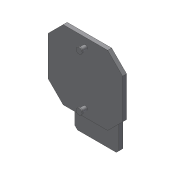
# Autodesk Inventor part: Maker-Bot-Raspberry-Pi-Holder
Saved by Autodesk Inventor 2015 (Build 190159000, 159)
## iProperties
Created: 2017-01-17
Part Number: Maker-Bot-Raspberry-Pi-Holder
Material: Generic
Document SubType Name: Modeling
Designer: Ghassan Yusuf
Density: 1 g/cm^3
Appearance: Default
Author: Ghassan Yusuf
Autodesk Inventor part; units mm, degrees
ref_plane "YZ Plane" through (0, 0, 0) normal (1, 0, 0) x (0, 1, 0)
ref_plane "XZ Plane" through (0, 0, 0) normal (0, 1, 0) x (-1, 0, 0)
ref_plane "XY Plane" through (0, 0, 0) normal (0, 0, 1) x (1, 0, 0)
sketch "Sketch1" plane through (0, 0, 0) normal (0, 1, 0) x (-1, 0, 0)
  line L0 (16.85, -26.3137) -> (-16.85, -26.3137)
  line L1 (-16.85, -26.3137) -> (-28.1637, -15)
  line L2 (-28.1637, -15) -> (-28.1637, 15)
  line L3 (-28.1637, 15) -> (-16.85, 26.3137)
  line L4 (-16.85, 26.3137) -> (16.85, 26.3137)
  line L5 (16.85, 26.3137) -> (28.1637, 15)
  line L6 (28.1637, 15) -> (28.1637, -15)
  line L7 (28.1637, -15) -> (16.85, -26.3137)
  point P0 (0, 0)
  point P1 (0, -26.3137)
  point P2 (28.1637, 0)
  point P3 (-28.1637, 0)
  point P4 (0, 26.3137)
  dimension "d2" = 30
  dimension "d6" = 16
  dimension "d7" = 16
  dimension "d9" = 16
  dimension "d10" = 16
  dimension "d11" = 135
  dimension "d12" = 135
  dimension "d13" = 135
  dimension "d14" = 135
  dimension "d15" = 30
  dimension "d16" = 33.7
  dimension "d17" = 33.7
  constraints: 16 end point, 4 midpoint, 3 perpendicular, 2 horizontal alignment, 2 parallel, 2 vertical alignment, 1 horizontal
  measures "d2" distance of L1.end L2.end
  measures "d6" distance of L4.end L5.end
  measures "d7" distance of L6.end L0.start
  measures "d9" distance of L2.end L3.end
  measures "d10" distance of L0.end L1.end
  measures "d11" angle of L0 L7
  measures "d12" angle of L1 L0
  measures "d13" angle of L4 L5
  measures "d14" angle of L4 L3
  measures "d15" distance of L5.end L6.end
  measures "d16" distance of L0.start L0.end
  measures "d17" distance of L3.end L4.end
extrude "Extrusion1" add sketch "Sketch1" along normal mid plane 3
sketch "Sketch2" plane through (0, 1.5, 0) normal (0, 1, 0) x (1, 0, 0)
  line L0 (-16.7, 23.8137) -> (16.7, 23.8137)
  line L1 (16.7, 23.8137) -> (16.7, 20.8137)
  line L2 (16.7, 20.8137) -> (-16.7, 20.8137)
  line L3 (-16.7, 20.8137) -> (-16.7, 23.8137)
  line L4 (16.85, 26.3137) -> (-16.85, 26.3137) projected
  point P0 (0, 0)
  point P1 (0, 23.8137)
  point P2 (0, 26.3137)
  dimension "d20" = 33.4
  dimension "d21" = 3
  dimension "d22" = 2.5
  constraints: 8 end point, 2 midpoint, 2 parallel, 1 horizontal, 1 perpendicular, 1 vertical alignment
  measures "d20" distance of L1.end L2.end
  measures "d21" distance of L0.end L1.end
  measures "d22" distance between parallel lines of L0 L4
extrude "Extrusion2" add sketch "Sketch2" along normal blind 5.7
sketch "Sketch4" plane through (0, 7.2, 0) normal (0, 1, 0) x (1, 0, 0)
  line L0 (-16.7, 12.2137) -> (16.7, 12.2137)
  line L1 (16.7, 12.2137) -> (16.7, 46.1137)
  line L2 (16.7, 46.1137) -> (-16.7, 46.1137)
  line L3 (-16.7, 46.1137) -> (-16.7, 12.2137)
  line L4 (-16.7, 23.8137) -> (-16.7, 20.8137) projected
  line L5 (16.7, 20.8137) -> (16.7, 23.8137) projected
  line L6 (-16.7, 20.8137) -> (16.7, 20.8137) projected
  line L7 (16.7, 23.8137) -> (-16.7, 23.8137) projected
  point P0 (0, 0)
  dimension "d25" = 8.6
  dimension "d26" = 22.3
  constraints: 8 end point, 2 collinear, 2 parallel, 1 horizontal, 1 perpendicular
  measures "d25" distance between parallel lines of L6 L0
  measures "d26" distance between parallel lines of L2 L7
extrude "Extrusion3" add sketch "Sketch4" along normal blind 3
chamfer "Chamfer1" distance 2 angle 45 4 edges at (-16.7, 8.7, -46.1137) (16.7, 8.7, -46.1137) (-16.7, 8.7, -12.2137) (16.7, 8.7, -12.2137)
sketch "Sketch5" plane through (0, -1.5, 0) normal (0, -1, 0) x (1, 0, 0)
  circle A0 centre (0, -20) radius 1.5
  circle A1 centre (0, 20) radius 1.5
  line L0 (-28.1637, -15) -> (-28.1637, 15) projected
  line L1 (-28.1637, 18.5) -> (28.1637, 18.5)
  line L2 (28.1637, -15) -> (28.1637, 15) projected
  line L3 (-28.1637, -18.5) -> (28.1637, -18.5)
  line L4 (-28.1637, 21.5) -> (28.1637, 21.5)
  line L5 (-28.1637, -21.5) -> (28.1637, -21.5)
  point P0 (0, 0)
  dimension "d34" = 3
  dimension "d35" = 3
  dimension "d42" = 43
  dimension "d43" = 21.5
  dimension "d44" = 37
  dimension "d45" = 18.5
  constraints: 8 end point, 3 parallel, 2 centre point, 2 point on line, 2 tangent, 1 horizontal
  measures "d34" diameter of A0
  measures "d35" diameter of A1
  measures "d42" distance between parallel lines of L5 L4
  measures "d43" distance from line of point (0, 0) L4
  measures "d44" distance between parallel lines of L3 L1
  measures "d45" distance from line of point (0, 0) L1
extrude "Extrusion4" add sketch "Sketch5" along normal blind 4
sketch "Sketch6" plane through (0, -5.5, -20) normal (0, -1, 0) x (1, 0, 0)
  circle A0 centre (0, 0) radius 1.5 projected
  circle A1 centre (0, 0) radius 2.25
  circle A2 centre (0, 40) radius 1.5 projected
  circle A3 centre (0, 40) radius 2.25
  point P0 (0, 20)
  dimension "d38" = 4.5
  dimension "d39" = 4.5
  constraints: 2 centre point, 2 coincident
  measures "d38" diameter of A1
  measures "d39" diameter of A3
extrude "Extrusion5" add sketch "Sketch6" along normal blind 0.8 contours A0 | A1 | A2 | A3
equation "\"d2\" = d0"
equation "\"d35\" = d34"
equation "\"d43\" = 0.5 * d42"
equation "\"d45\" = 0.5 * d44"
equation "\"d39\" = d38"
equation "\"d0\" = 30"
body "Solid1"
